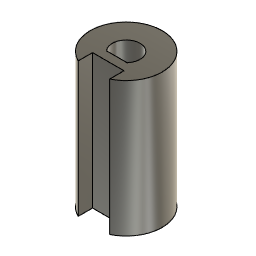
N20_BT09_ShaftAdapter v6 (Autodesk Fusion 360 design; units mm, degrees)
Autodesk Fusion 360 part; units mm, degrees
cylinder "CylinderPrimitive1" add diameter 8 height 15 placed x (1, 0, 0) y (0, 1, 0) z (0, 0, 1) at (0, 0, 0)
hole "Hole1" at (0, 0, 15) direction (0, 0, -1) diameter 3.1 depth 18 tip angle 118
box "BoxPrimitive2" add length 0.45 width 2.9 height 20 placed x (0, 1, 0) y (-1, 0, 0) z (0, 0, 1) at (1.4, -1.5503, 0)
extrude "Extrude1" cut 1 faces at (-0.5333, -1.4003, 20) along direction (0, 0, -1) blind 5
extrude "Extrude2" add 1 faces at (0.3639, -1.1003, 5) along direction (0, 1, 0) blind 0.05
extrude "Extrude3" add 1 faces at (1.0917, -1.0836, 10) along direction (1, 0, 0) blind 0.14
extrude "Extrude4" add 1 faces at (-1.0917, -1.0836, 10) along direction (-1, 0, 0) blind 0.14
box "BoxPrimitive3" cut length 2 width 3.5 height 17 placed x (0, 1, 0) y (-1, 0, 0) z (0, 0, 1) at (1.75, -4, 0)
